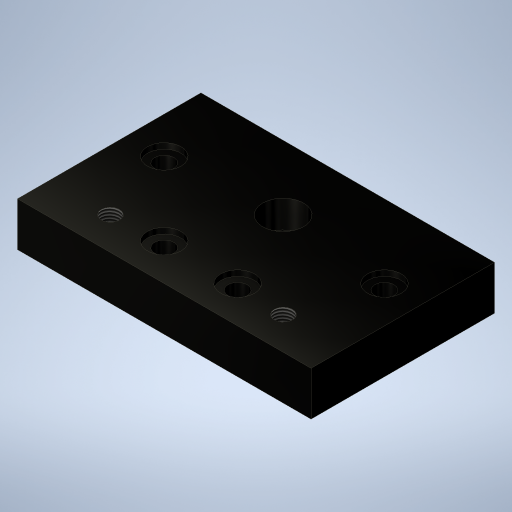
# Autodesk Inventor part: C-Beam End Mount
Saved by Autodesk Inventor 2024.2 (Build 282272000, 272)
## iProperties
Created: 2020-11-22
Part Number: C-Beam End Mount
Material: Aluminum 6061
Document SubType Name: Modeling
Designer: asus
Density: 2.7 g/cm^3
Appearance: Gunmetal
Author: asus
Autodesk Inventor part; units mm, degrees
ref_plane "YZ Plane" through (0, 0, 0) normal (1, 0, 0) x (0, 1, 0)
ref_plane "XZ Plane" through (0, 0, 0) normal (0, 1, 0) x (-1, 0, 0)
ref_plane "XY Plane" through (0, 0, 0) normal (0, 0, 1) x (1, 0, 0)
sketch "Sketch1" plane through (0, 0, 0) normal (0, 1, 0) x (-1, 0, 0)
  line L0 (40, -25) -> (-40, -25)
  line L1 (-40, -25) -> (-40, 25)
  line L2 (-40, 25) -> (40, 25)
  line L3 (40, 25) -> (40, -25)
  circle A0 centre (30, -5) radius 2.6
  circle A1 centre (0, -7.4) radius 5.59
  circle A2 centre (-30, -5) radius 2.6
  circle A3 centre (10, 15) radius 2.6
  circle A4 centre (-10, 15) radius 2.6
  circle A5 centre (23.57, 16.1) radius 2.5
  circle A6 centre (-23.57, 16.1) radius 2.5
  point P0 (40, 0)
  point P1 (0, 0)
  point P2 (0, -25)
  dimension "d3" = 80
  dimension "d4" = 50
  dimension "d5" = 5.2
  dimension "d6" = 5.2
  dimension "d7" = 5
  dimension "d8" = 11.18
  dimension "d9" = 10
  dimension "d10" = 10
  dimension "d11" = 30
  dimension "d12" = 30
  dimension "d13" = 10
  dimension "d14" = 30
  dimension "d15" = 30
  dimension "d16" = 10
  dimension "d17" = 40
  dimension "d18" = 32.4
  dimension "d19" = 8.9
  dimension "d20" = 8.9
  dimension "d21" = 16.43
  dimension "d44" = 16.43
  constraints: 8 end point, 7 centre point, 3 equal radius, 2 midpoint, 2 parallel, 1 horizontal, 1 horizontal alignment, 1 perpendicular, 1 vertical alignment
  measures "d3" distance of L1.end L2.end
  measures "d4" distance of L0.end L1.end
  measures "d5" diameter of A0
  measures "d6" diameter of A2
  measures "d7" diameter of A5
  measures "d8" diameter of A1
  measures "d9" distance from line of L3 A0.centre
  measures "d10" distance from line of L1 A2.centre
  measures "d11" distance from line of L2 A0.centre
  measures "d12" distance from line of L2 A2.centre
  measures "d13" distance from line of L2 A3.centre
  measures "d14" distance from line of L3 A3.centre
  measures "d15" distance from line of L1 A4.centre
  measures "d16" distance from line of L2 A4.centre
  measures "d17" distance from line of L3 A1.centre
  measures "d18" distance from line of L2 A1.centre
  measures "d19" distance from line of L2 A5.centre
  measures "d20" distance from line of L2 A6.centre
  measures "d21" distance from line of L3 A5.centre
  measures "d44" distance from line of L1 A6.centre
extrude "Extrusion1" add sketch "Sketch1" along normal blind 12
sketch "Sketch2" plane through (0, 12, 0) normal (0, 1, 0) x (1, 0, 0)
  circle A0 centre (-30, 5) radius 2.6 projected
  circle A1 centre (-10, -15) radius 2.6 projected
  circle A2 centre (10, -15) radius 2.6 projected
  circle A3 centre (30, 5) radius 2.6 projected
  circle A4 centre (-30, 5) radius 4.6
  circle A5 centre (-10, -15) radius 4.6
  circle A6 centre (10, -15) radius 4.6
  circle A7 centre (30, 5) radius 4.6
  point P0 (0, 0)
  dimension "d25" = 9.2
  constraints: 4 centre point, 4 coincident, 3 equal radius
  measures "d25" diameter of A4
extrude "Extrusion2" cut sketch "Sketch2" against normal blind 1.55 contours A3 | A4 | A5 | A6 | A7
thread "Thread1" size "M5x0.8" class "6H" standard "ANSI Metric M Profile" full length
thread "Thread2" size "M5x0.8" class "6H" standard "ANSI Metric M Profile" full length
sketch "Sketch3" plane through (0, 0, 0) normal (0, -1, 0) x (1, 0, 0)
  circle A0 centre (0, -7.4) radius 5.59 projected
  circle A1 centre (0, -7.4) radius 8.05
  point P0 (0, 0)
  dimension "d32" = 16.1
  constraints: 1 centre point, 1 coincident
  measures "d32" diameter of A1
extrude "Extrusion3" cut sketch "Sketch3" against normal blind 4.5 contours A0 | A1
sketch "Sketch4" plane through (40, 0, -25) normal (0, 0, -1) x (-1, 0, 0)
  line L0 (0, 0) -> (0, 12) projected
  point P0 (40, 0)
  point P1 (30, 6)
  point P2 (50, 6)
  point P3 (0, 6)
  dimension "d35" = 30
  dimension "d36" = 20
  constraints: 2 horizontal alignment, 1 midpoint
  measures "d35" distance from line of L0 point (30, 6)
  measures "d36" distance of point (50, 6) point (30, 6)
hole "Hole1" at (10, 6, -25) at (-10, 6, -25) direction (0, 0, 1) diameter 4.134 depth 10 thread size "M5x0.8" class "6H" standard "ISO Metric profile"
body "Solid1"
